Autodesk Fusion 360 part; units mm, degrees
(part 2 of 2)
  spline S71 degree 3 poles (-117.0389, -62.1859) (-117.0887, -62.1627) (-117.1897, -62.1158) (-117.2558, -62.0262) (-117.2893, -61.9808) knots 0 0 0 0 0.016202 0.032838 0.032838 0.032838 0.032838
  spline S72 degree 3 poles (-117.2893, -61.9808) (-117.3167, -61.929) (-117.3726, -61.8232) (-117.3796, -61.7035) (-117.3831, -61.6424) knots 0 0 0 0 0.017346 0.035479 0.035479 0.035479 0.035479
  spline S73 degree 3 poles (-117.3831, -61.6424) (-117.3781, -61.5663) (-117.3683, -61.4194) (-117.2824, -61.3001) (-117.241, -61.2425) knots 0 0 0 0 0.022366 0.043205 0.043205 0.043205 0.043205
  spline S74 degree 3 poles (-117.241, -61.2425) (-117.1845, -61.1947) (-117.0613, -61.0905) (-116.9022, -61.0608) (-116.8162, -61.0448) knots 0 0 0 0 0.021852 0.047577 0.047577 0.047577 0.047577
  spline S75 degree 3 poles (-116.8162, -61.0448) (-116.8602, -61.0176) (-116.9439, -60.966) (-117.0142, -60.8972) (-117.0476, -60.8646) knots 0 0 0 0 0.015439 0.029411 0.029411 0.029411 0.029411
  spline S76 degree 3 poles (-117.0476, -60.8646) (-117.0845, -60.8198) (-117.1753, -60.7095) (-117.2505, -60.5881) (-117.2952, -60.5159) knots 0 0 0 0 0.017387 0.0428 0.0428 0.0428 0.0428
  line L200 (-117.2952, -60.5159) -> (-117.5574, -60.097)
  line L201 (-117.5574, -60.097) -> (-117.0389, -60.097)
  line L202 (-117.0389, -60.097) -> (-116.7254, -60.5643)
  spline S77 degree 3 poles (-116.7254, -60.5643) (-116.6799, -60.6333) (-116.6085, -60.7418) (-116.5266, -60.8426) (-116.4969, -60.8792) knots 0 0 0 0 0.024776 0.038931 0.038931 0.038931 0.038931
  spline S78 degree 3 poles (-116.4969, -60.8792) (-116.4768, -60.8992) (-116.4387, -60.9369) (-116.3897, -60.9584) (-116.3665, -60.9686) knots 0 0 0 0 0.008409 0.015927 0.015927 0.015927 0.015927
  spline S79 degree 3 poles (-116.3665, -60.9686) (-116.337, -60.9758) (-116.2654, -60.9933) (-116.1916, -60.9934) (-116.1482, -60.9935) knots 0 0 0 0 0.009093 0.022035 0.022035 0.022035 0.022035
  line L203 (-116.1482, -60.9935) -> (-116.0603, -60.9935)
  line L204 (-133.0002, -61.8812) -> (-133.0002, -60.097)
  line L205 (-133.0002, -60.097) -> (-132.5666, -60.097)
  line L206 (-131.9294, -62.2445) -> (-133.6359, -62.2445)
  line L207 (-133.6359, -62.2445) -> (-133.6359, -61.8812)
  line L208 (-133.6359, -61.8812) -> (-133.0002, -61.8812)
  arc A24 (-121.5415, -56.616) -> (-121.5415, -53.538) centre (-118.398, -55.077) ccw
  arc A25 (-121.5415, -53.538) -> (-121.5415, -56.616) centre (-124.685, -55.077) ccw
  line L209 (-127.6945, -62.2445) -> (-126.9255, -60.097)
  line L210 (-126.9255, -60.097) -> (-126.4626, -60.097)
  line L211 (-126.4626, -60.097) -> (-125.695, -62.2445)
  line L212 (-125.695, -62.2445) -> (-126.1652, -62.2445)
  line L213 (-126.1652, -62.2445) -> (-126.7087, -60.6551)
  line L214 (-126.7087, -60.6551) -> (-127.2346, -62.2445)
  line L215 (-127.2346, -62.2445) -> (-127.6945, -62.2445)
  line L216 (-129.549, -60.4588) -> (-129.549, -60.097)
  line L217 (-129.549, -60.097) -> (-127.9157, -60.097)
  line L218 (-127.9157, -60.097) -> (-127.9157, -62.2445)
  line L219 (-127.9157, -62.2445) -> (-129.508, -62.2445)
  line L220 (-129.508, -62.2445) -> (-129.508, -61.8812)
  line L221 (-129.508, -61.8812) -> (-128.3493, -61.8812)
  line L222 (-128.3493, -61.8812) -> (-128.3493, -61.4051)
  line L223 (-128.3493, -61.4051) -> (-129.4274, -61.4051)
  line L224 (-129.4274, -61.4051) -> (-129.4274, -61.0433)
  line L225 (-129.4274, -61.0433) -> (-128.3493, -61.0433)
  line L226 (-128.3493, -61.0433) -> (-128.3493, -60.4588)
  line L227 (-128.3493, -60.4588) -> (-129.549, -60.4588)
  line L228 (-132.5666, -60.097) -> (-132.5666, -61.8812)
  line L229 (-132.5666, -61.8812) -> (-131.9294, -61.8812)
  line L230 (-131.9294, -61.8812) -> (-131.9294, -62.2445)
  line L231 (-130.3239, -61.4974) -> (-130.3239, -60.097)
  line L232 (-130.3239, -60.097) -> (-129.9211, -60.097)
  line L233 (-129.9211, -60.097) -> (-129.9211, -62.2445)
  line L234 (-129.9211, -62.2445) -> (-130.3429, -62.2445)
  line L235 (-130.3429, -62.2445) -> (-131.2219, -60.8104)
  line L236 (-131.2219, -60.8104) -> (-131.2219, -62.2445)
  line L237 (-131.2219, -62.2445) -> (-131.6247, -62.2445)
  line L238 (-131.6247, -62.2445) -> (-131.6247, -60.097)
  line L239 (-131.6247, -60.097) -> (-131.1896, -60.097)
  line L240 (-131.1896, -60.097) -> (-130.3239, -61.4974)
  dimension "d100" = 3
  dimension "d101" = 5
  dimension "d102" = 5
  dimension "d103" = 10
  dimension "d104" = 10
  dimension "d105" = 5
  dimension "d106" = 5
  dimension "d107" = 5
  dimension "d108" = 5
  dimension "d109" = 5
  dimension "d110" = 5
  dimension "d111" = 5
  dimension "d112" = 5
  dimension "d113" = 60
  dimension "d114" = 1
  dimension "d115" = 1
  constraint horizontal L26
  constraint vertical L27
  constraint horizontal L28
  constraint vertical L29
  constraint horizontal L30
  constraint vertical L31
  constraint horizontal L32
  constraint vertical L33
  constraint tangent L26 A8
  constraint tangent L31 A12
  constraint tangent L28 A15
  constraint tangent L29 A8
  constraint tangent L29 A15
  constraint tangent L28 A14
  constraint tangent L26 A9
  constraint tangent L33 A10
  constraint tangent L27 A9
  constraint tangent L33 A13
  constraint tangent L27 A14
  constraint tangent L32 A13
  constraint tangent L32 A12
  constraint tangent L30 A11
  constraint tangent L31 A11
  constraint tangent L30 A10
  constraint collinear L26 L30
  constraint collinear L28 L32
  measures "d100" distance of L25 L26
  measures "d101" distance of L23 L28
  measures "d102" distance of L27 L33
  measures "d103" distance of L22 L29
  measures "d104" distance of L24 L31
  measures "d105" radius of A15
  measures "d106" radius of A8
  measures "d107" radius of A9
  measures "d108" radius of A14
  measures "d109" radius of A13
  measures "d110" radius of A12
  measures "d111" radius of A10
  measures "d112" radius of A11
  measures "d113" distance of L27 L29
extrude "Extrude5" cut sketch "Sketch6" against normal blind 0.5 contours L26 L27 L28 L29 A8 A9 A14 A15 | L30 L31 L32 L33 A10 A11 A12 A13
sketch "Sketch7" plane through (0, 0, 1.5) normal (0, 0, 1) x (-1, 0, 0)
  line L0 (-13, -8) -> (-41.4668, -8) construction
  line L1 (-41.4668, -8) -> (-41.4668, -14) construction
  line L2 (-41.4668, -14) -> (-13, -14) construction
  line L3 (-13, -14) -> (-13, -8) construction
  line L4 (-11, -10) -> (-11, -90)
  line L5 (-65, -6) -> (-15, -6)
  line L6 (-114.5585, -86) -> (-135, -86) construction
  line L7 (-135, -86) -> (-135, -92) construction
  line L8 (-135, -92) -> (-114.5585, -92) construction
  line L9 (-114.5585, -92) -> (-114.5585, -86) construction
  line L10 (-76, -10) -> (-76, -90)
  line L11 (-133, -6) -> (-80, -6)
  line L12 (-133, -94) -> (-80, -94)
  line L13 (-137, -10) -> (-137, -90)
  dimension "d139" = 6
  dimension "d140" = 2
  dimension "d141" = 2
  dimension "d144" = 6
  dimension "d196" = 2
  dimension "d197" = 2
  text T0 "PACEMAKER" font "Arial" height 6 bold align ink ink in box 0 x 0 at (-13, -8) x (-1, 0) y (0, -1) spacing 1 height is em
  text T1 "HEART" font "Arial" height 6 bold align ink ink in box 0 x 0 at (-114.5585, -86) x (-1, 0) y (0, -1) spacing 1 height is em
  constraint perpendicular L0 L1
  constraint parallel L0 L2
  constraint parallel L1 L3
  constraint perpendicular L6 L7
  constraint parallel L6 L8
  constraint parallel L7 L9
  measures "d139" distance of L0.start L2.end
  measures "d140" distance of L3 L4
  measures "d141" distance of L0 L5
  measures "d144" distance of L6.start L8.end
  measures "d196" distance of L8 L12
  measures "d197" distance of L7 L13
extrude "Extrude6" cut sketch "Sketch7" against normal blind 0.5 text T0 T1
equation "d10 = d76"
equation "d11 = d76"
equation "d15 = d96 / 2"
equation "d27 = d26"
equation "d34 = d5"
equation "d35 = d5"
equation "d36 = d5"
equation "d37 = d26"
equation "d38 = d26"
equation "d39 = d26"
equation "d40 = d26"
equation "d41 = d26"
equation "d42 = d26"
equation "d45 = d158"
equation "d46 = d158"
equation "d96 = 8.666174 mm"
equation "d97 = d11 / 2"
equation "d98 = d97"
equation "d99 = d97"
equation "d106 = d105"
equation "d107 = d105"
equation "d108 = d105"
equation "d109 = d105"
equation "d110 = d105"
equation "d111 = d105"
equation "d112 = d105"
equation "d154 = d153 / 2"
equation "d157 = d158"
equation "d163 = d76"
equation "d179 = d178"
equation "d180 = d178"
equation "d196 = d141"
equation "d197 = d140"
equation "d202 = ( ( ( d190 - d132 + 4 mm ) / 2 mm ) * 1 mm )"
equation "d203 = ( d192 - d135 + 4 mm ) / 2"
equation "d220 = ( d210 - d124 + 4 mm ) / 2"
equation "d221 = ( d214 - d126 + 4 mm ) / 2"
equation "d245 = 1.295 mm + ( 2.54 / 2 ) * 1 mm"
equation "d248 = d239"
